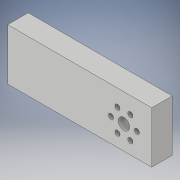
# Autodesk Inventor part: MotorHolderA
Saved by Autodesk Inventor 2017 (Build 210142000, 142)
## iProperties
Created: 2017-12-08
Part Number: MotorHolderA
Material: Generic
Document SubType Name: Modeling
Designer: User
Density: 1 g/cm^3
Appearance: Default
Author: User
Autodesk Inventor part; units mm, degrees
ref_plane "YZ Plane" through (0, 0, 0) normal (1, 0, 0) x (0, 1, 0)
ref_plane "XZ Plane" through (0, 0, 0) normal (0, 1, 0) x (-1, 0, 0)
ref_plane "XY Plane" through (0, 0, 0) normal (0, 0, 1) x (1, 0, 0)
sketch "Sketch1" plane through (0, 0, 0) normal (0, 0, 1) x (1, 0, 0)
  line L0 (0, 0) -> (63.5, 0)
  line L1 (0, 0) -> (63.5, 0)
  line L2 (63.5, 0) -> (63.5, 31.75)
  line L3 (63.5, 31.75) -> (0, 31.75)
  line L4 (0, 31.75) -> (0, 0)
  dimension "d0" = 63.5
  dimension "d1" = 31.75
  constraints: 10 end point, 2 horizontal, 2 parallel, 1 perpendicular
  measures "d0" distance of L0.start L0.end
  measures "d1" distance of L2.end L1.end
extrude "Extrusion1" add sketch "Sketch1" along normal blind 19.05
sketch "Sketch2" plane through (0, 0, 19.05) normal (0, 0, 1) x (1, 0, 0)
  line L0 (63.5, 0) -> (63.5, 31.75) projected
  line L1 (63.5, 7.8489) -> (80.6196, 7.8489) construction
  line L2 (46.3804, 0) -> (46.3804, 14.605)
  circle A0 centre (46.3804, 14.605) radius 3.4925
  circle A1 centre (46.3804, 14.605) radius 8.001
  circle A2 centre (54.3814, 14.605) radius 1.5875
  circle A3 centre (50.3809, 21.5341) radius 1.5875
  circle A4 centre (46.3804, 14.605) radius 8.001
  circle A5 centre (42.3799, 21.5341) radius 1.5875
  circle A6 centre (46.3804, 14.605) radius 8.001
  circle A7 centre (38.3794, 14.605) radius 1.5875
  circle A8 centre (46.3804, 14.605) radius 8.001
  circle A9 centre (42.3799, 7.6759) radius 1.5875
  circle A10 centre (46.3804, 14.605) radius 8.001
  circle A11 centre (50.3809, 7.6759) radius 1.5875
  circle A12 centre (46.3804, 14.605) radius 8.001
  point P0 (0, 0)
  dimension "d9" = 16.002
  dimension "d6" = 14.605
  dimension "d7" = 6.985
  dimension "d17" = 3.175
  dimension "d20" = 360
  dimension "d61" = 17.1196
  constraints: 7 centre point, 4 end point, 2 coincident, 2 horizontal alignment, 1 horizontal, 1 point on line, 41 other
  measures "d6" distance of L2.start L2.end
  measures "d7" diameter of A0
  measures "d17" diameter of A2
  measures "d61" distance from line of L0 L2.end
extrude "Extrusion2" cut sketch "Sketch2" against normal blind 19.05 contours A0 | A1 A2 | A1 A2 | A3 A1 | A1 A3 | A11 A1 | A1 A11 | A5 A1 | A1 A5 | A9 A1 | A1 A9 | A7 A1 | A1 A7
thicken "Thicken1" operation add thickness 25.4 both sides no extend neighbours yes toward (-1, 0, 0) faces at (0, 21.1667, 12.7)
thicken "Thicken2" operation add thickness 3.175 both sides no extend neighbours yes toward (0, 0, -1) faces at (-4.6694, 15.4517, 19.05)
thicken "Thicken3" operation add thickness 3.175 both sides no extend neighbours yes toward (0, 0, -1) faces at (-4.6694, 15.4517, 15.875)
sketch "Sketch5" plane through (-25.4, 0, 0) normal (0, -1, 0) x (1, 0, 0)
  line L0 (0, 0) -> (0, 12.7) projected
  line L1 (88.9, 0) -> (88.9, 12.7) projected
  line L2 (0, 0) -> (88.9, 0) projected
  point P0 (25.4, 0)
  point P1 (6.35, 6.35)
  point P2 (44.45, 6.35)
  point P3 (82.55, 6.35)
  dimension "d57" = 6.35
  dimension "d58" = 44.45
  dimension "d59" = 88.9
  dimension "d60" = 6.35
  measures "d57" distance from line of L1 point (82.55, 6.35)
  measures "d58" distance from line of L1 point (44.45, 6.35)
  measures "d59" distance of L1.end L0.end
  measures "d60" distance from line of L0 point (6.35, 6.35)
hole "Hole1" at (-19.05, 0, 6.35) at (19.05, 0, 6.35) at (57.15, 0, 6.35) direction (0, 1, 0) diameter 3.302 depth 7.62 tip angle 118 thread size "8-32 UNC" class "2B" standard "ANSI Unified Screw Threads"
equation "\"d58\" = 0.5 * d59"
body "Solid1"
